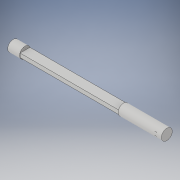
# Autodesk Inventor part: Cheville
Saved by Autodesk Inventor 2019 (Build 230136000, 136)
## iProperties
Created: 2020-01-16
Part Number: Cheville
Material: Générique
Document SubType Name: Modeling
Designer: Quentin
Density: 1 g/cm^3
Appearance: Par défaut
Author: Quentin
Autodesk Inventor part; units mm, degrees
ref_plane "YZ Plane" through (0, 0, 0) normal (1, 0, 0) x (0, 1, 0)
ref_plane "XZ Plane" through (0, 0, 0) normal (0, 1, 0) x (-1, 0, 0)
ref_plane "XY Plane" through (0, 0, 0) normal (0, 0, 1) x (1, 0, 0)
sketch "Esquisse1" plane through (0, 0, 0) normal (0, 0, 1) x (1, 0, 0)
  line L0 (0, 10) -> (5, 10)
  line L1 (5, 6) -> (5, 10)
  line L2 (5, 6) -> (55, 6)
  line L3 (55, 6) -> (55, 10)
  line L4 (55, 0) -> (55, 4)
  line L5 (55, 4) -> (5, 4)
  line L6 (5, 6) -> (5, 4)
  line L7 (55, 6) -> (55, 4)
  point P0 (0, 0)
  point P1 (25, 10)
  dimension "d39" = 50
  dimension "d40" = 5
  constraints: 16 end point, 2 point on line, 1 horizontal, 1 parallel, 1 perpendicular, 1 vertical
  measures "d39" distance of L1.start L2.end
  measures "d40" distance of L0.start L0.end
extrude "Extrusion1" add sketch "Esquisse1" along normal blind 5
sketch "Esquisse9" plane through (5, 6, 0) normal (0, 1, 0) x (1, 0, 0)
  line L0 (0, 0) -> (5, 0)
  line L1 (5, 0) -> (45, 0)
  line L2 (0, 0) -> (50, 0) projected
  line L3 (45, 0) -> (45, -2.5)
  line L4 (5, 0) -> (5, -2.5)
  circle A0 centre (5, -2.5) radius 1
  circle A1 centre (45, -2.5) radius 1
  point P0 (-5, 0)
  dimension "d42" = 5
  dimension "d43" = 40
  dimension "d44" = 2
  dimension "d45" = 2
  constraints: 8 end point, 2 centre point, 2 coincident, 1 perpendicular, 1 point on line, 1 vertical
  measures "d42" distance of L0.start L0.end
  measures "d43" distance of L0.end L1.end
  measures "d44" diameter of A0
  measures "d45" diameter of A1
extrude "Extrusion9" add sketch "Esquisse9" against normal blind 3
sketch "Esquisse10" plane through (55, 4, 0) normal (1, 0, 0) x (0, 0, -1)
  line L0 (0, 0) -> (0, 2) projected
  line L1 (0, 1) -> (-5, 1)
  line L2 (-5, 0) -> (-5, 2) projected
  circle A0 centre (-2.5, 1) radius 2.75
  point P0 (0, -4)
  dimension "d50" = 5.5
  constraints: 3 midpoint, 2 end point, 1 centre point
  measures "d50" diameter of A0
extrude "Extrusion10" add sketch "Esquisse10" along normal blind 22
sketch "Esquisse11" plane through (5, 4, 0) normal (-1, 0, 0) x (0, 0, 1)
  circle A0 centre (2.5, 1) radius 2.75 projected
  circle A1 centre (2.5, 1) radius 2.75
  point P0 (0, -4)
  constraints: 1 centre point, 1 coincident
extrude "Extrusion11" add sketch "Esquisse11" along normal blind 6
sketch "Esquisse14" plane through (0, 0, 5) normal (0, 0, 1) x (1, 0, 0)
  line L0 (55, 4) -> (55, 6) projected
  line L1 (55, 5) -> (73.9, 5)
  circle A0 centre (73.9, 5) radius 1
  point P0 (0, 0)
  dimension "d59" = 18.9
  dimension "d60" = 2
  constraints: 2 end point, 1 centre point, 1 coincident, 1 horizontal, 1 midpoint
  measures "d59" distance of L1.start L1.end
  measures "d60" diameter of A0
extrude "Extrusion12" cut sketch "Esquisse14" against normal through all
